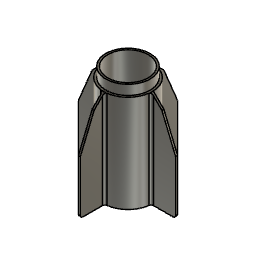
Big Fin Assembly v2 (Autodesk Fusion 360 design; units mm, degrees)
Autodesk Fusion 360 part; units mm, degrees
sketch "Sketch1" plane through (0, 0, 0) normal (0, 0, 1) x (1, 0, 0)
  line L0 (0.508, 25.4) -> (0.5099, 12.6898)
  line L1 (-0.5117, -25.4) -> (-0.5117, -12.6897)
  circle A0 centre (0, 0) radius 12.7
  line L2 (-12.6897, -0.5117) -> (-25.4, -0.5117)
  line L3 (12.6897, 0.5117) -> (25.4, 0.5117)
  line L4 (-0.5099, 12.6898) -> (-0.508, 25.4)
  line L5 (-25.4, 0.5117) -> (-25.4, -0.5117)
  circle A1 centre (0, 0) radius 11.557
  line L6 (0.5117, -25.4) -> (-0.5117, -25.4)
  line L7 (-25.4, 0.5117) -> (-12.6897, 0.5117)
  line L8 (0.5117, -12.6897) -> (0.5117, -25.4)
  line L9 (-0.508, 25.4) -> (0.508, 25.4)
  line L10 (25.4, 0.5117) -> (25.4, -0.5117)
  line L11 (1.016, 25.521) -> (0, 25.521)
  line L12 (25.4, -0.5117) -> (12.6897, -0.5117)
  circle A2 centre (0, 0) radius 10.5519
  dimension "d2" = -1.143
  dimension "d1" = 25.4
  dimension "d8" = 1.016
  constraint coincident A0.centre A1.centre
  constraint horizontal L11
  constraint perpendicular L10 L12
  constraint coincident L4.start A0
  constraint coincident L0.end A0
  constraint coincident L7.end A0
  constraint coincident L2.start A0
  constraint coincident L12.end A0
  constraint coincident L3.start A0
  constraint coincident L8.start A0
  constraint coincident L1.end A0
  constraint concentric A0 A2
  measures "d1" diameter of A0
  measures "d8" distance of L4.end L0.start
extrude "Extrude2" add sketch "Sketch1" along normal blind 55.88 contours A1 makes body 1
extrude "Extrude1" add sketch "Sketch1" along normal blind 50.8 separate body contours L0 A0 L4 L9 | A0 | A0 L3 L10 L12 | A0 L2 L5 L7 | L1 A0 L6 L8 makes body 2
chamfer "Chamfer1" distance 12.7 angle 45 4 edges at (25.4, 0, 50.8) (0, -25.4, 50.8) (0, 25.4, 50.8) (-25.4, 0, 50.8) on bodies 2
chamfer "Chamfer2" distance 10.16 angle 45 4 edges at (25.4, 0, 38.1) (0, -25.4, 38.1) (-25.4, 0, 38.1) (0, 25.4, 38.1) on bodies 2
fillet "Fillet1" radius 1.27 6 edges at (-0.5099, 12.6898, 25.4) (-12.6897, 0.5117, 25.4) (-12.6897, -0.5117, 25.4) (-0.5117, -12.6897, 25.4) (0.5117, -12.6897, 25.4) (12.6897, -0.5117, 25.4) on bodies 2
fillet "Fillet2" radius 1.27 4 edges at (25.4, 0, 0) (0, 25.4, 0) (-25.4, 0, 0) (0, -25.4, 0) on bodies 2
